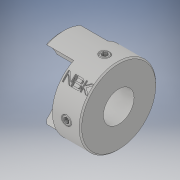
# Autodesk Inventor part: MJT-30-BL-8-12 Hub 2
Saved by Autodesk Inventor 2019 (Build 230136000, 136)
## iProperties
Created: 2023-09-29
Part Number: MJT-30-BL-8-12 Hub 2
Material: Generic
Catalog Web Link: www.cadenas.de
Description: MJT Hub 2-
Vendor: NBK
Document SubType Name: Modeling
Designer: psAdmin
Manufacturer: NBK
Mass: 7.813 g
Surface Area: 34.5036 cm^2
Volume: 7.813 cm^3
Density: 1 g/cm^3
Appearance: PSOLRGB-175-175-175
Category: PARTsolutions
Company: NBK
Title: MJT-30-BL-8-12 Hub 2
Author: Cadenas PARTsolutions
PSOL_IDENT_0: {$CADENAS_DATA/23d-libs/nbk/motion_control_parts/couplicon_mini/jaw_type/mjt/mjt_3.prj},187 {VTYP=3D
PSOL_IDENT_1: },{NB=MJT-30-BL-8-12 Hub 2},{LINA=MJT-30-BL-8-12 Hub 2},{NN=MJT Hub 2},{DATE=25.09.2023 00:41:45},{G
PSOL_IDENT_2: EOMDATE=30.03.2016 02:13:54},{VERSION=},{LINEID=30},{WBVAR=D1D2},{WBNUMERIC=}  {NB=MJT-30-BL-8-12 Hu
PSOL_IDENT_3: b 2},{LINA=MJT-30-BL-8-12 Hub 2},{KT=DUMMY},{CN=MJT-30-BL},{D1D2=8-12},{D1D2X1='6-6','6-6.35','6-7','
PSOL_IDENT_4: 6-8','6-9.525','6-10','6-11','6-12','6-14','6-15','6-16','6.35-6.35','6.35-7','6.35-8','6.35-9.525','
PSOL_IDENT_5: 6.35-10','6.35-11','6.35-12','6.35-14','6.35-15','6.35-16','7-7','7-8','7-9.525','7-10','7-11','7-12'
PSOL_IDENT_6: ,'7-14','7-15','7-16','8-8','8-9.525','8-10','8-11','8-12','8-14','8-15','8-16','9.525-9.525','9.525
PSOL_IDENT_7: -10','9.525-11','9.525-12','9.525-14','9.525-15','9.525-16','10-10','10-11','10-12','10-14','10-15','
PSOL_IDENT_8: 10-16','11-11','11-12','11-14','11-15','11-16','12-12','12-14','12-15','12-16','14-14','14-15','14-1
PSOL_IDENT_9: 6','15-15','15-16','16-16'},{VERS=1},{YV=0.5},{YU=1.0},{A=30},{L=11},{W=35},{B=10},{C=1.5},{F=5.5},{
PSOL_IDENT_10: M=M4},{KDMM=3.242},{NDM=4.00},{KDMV=3.141},{DV=7.00},{D1=8},{D2=12},{DP=13.22},{DP1=0.00},{RV=1.500}
PSOL_IDENT_11: ,{S=2.0}
NB: MJT-30-BL-8-12 Hub 2
NN: MJT Hub 2
NBSYN: $CN.-$D1D2. Hub 2
LINA: MJT-30-BL-8-12 Hub 2
CATALOG: NBK (Nabeya Bi-tech Kaisha
CN: MJT-30-BL
D1D2: 8-12
D1D2X1: '6-6','6-6.35','6-7','6-8','6-9.525','6-10','6-11','6-12','6-14','6-15','6-16','6.35-6.35','6.35-7','6.35-8','6.35-9.525','6.35-10','6.35-11','6.35-12','6.35-14','6.35-15','6.35-16','7-7','7-8','7-9.525','7-10','7-11','7-12','7-14','7-15','7-16','8-8','8-9.525','8-10','8-11','8-12','8-14','8-15','8-16','9.525-9.525','9.525-10','9.525-11','9.525-12','9.525-14','9.525-15','9.525-16','10-10','10-11','10-12','10-14','10-15','10-16','11-11','11-12','11-14','11-15','11-16','12-12','12-14','12-15','12-16','14-14','14-15','14-16','15-15','15-16','16-16'
VERS: 1
YV: 0.5
YU: 1
A: 30
L: 11
W: 35
B: 10
C: 1.5
F: 5.5
M: M4
KDMM: 3.242
NDM: 4
KDMV: 3.141
DV: 7
DP: 13.22
DP1: 0
RV: 1.5
S: 2
SUPPLIER: NBK
ARTICLENO: MJT-30-BL-8-12 Hub 2
BOMINFO: MJT-30-BL-8-12 Hub 2
CREATOR: CADENAS GmbH
Autodesk Inventor part; units mm, degrees
sketch "Sketch_1" plane through (0, 0, 0) normal (0, 1, 0) x (-1, 0, 0)
  line L0 (22.5, 0) -> (0, 0)
  line L1 (22.5, 14) -> (21.5, 15)
  line L2 (21.5, 15) -> (0.5, 15)
  line L3 (0.5, 15) -> (0, 14.5)
  line L4 (0, 14.5) -> (0, 6)
  line L5 (0, 6) -> (22.5, 6)
  line L6 (22.5, 6) -> (22.5, 14)
  constraints: 14 end point
revolve "Revolution1" add sketch "Sketch_1" angle 360 about axis through (-22.5, 0, 0) along (-1, 0, 0)
sketch "Sketch_2" plane through (-11, 0, 0) normal (1, 0, 0) x (0, 0, -1)
  arc A0 (-6.61, 13.4651) -> (-6.61, -13.4651) centre (0, 0) ccw
  arc A1 (-6.61, -13.4651) -> (-1.6525, -7.3157) centre (-17.0197, 0) ccw
  arc A2 (-1.6525, -7.3157) -> (1.6525, -7.3157) centre (0, 0) ccw
  arc A3 (1.6525, -7.3157) -> (6.61, -13.4651) centre (17.0197, 0) ccw
  arc A4 (6.61, -13.4651) -> (6.61, 13.4651) centre (0, 0) ccw
  arc A5 (6.61, 13.4651) -> (1.6525, 7.3157) centre (17.0197, 0) ccw
  arc A6 (1.6525, 7.3157) -> (-1.6525, 7.3157) centre (0, 0) ccw
  arc A7 (-1.6525, 7.3157) -> (-6.61, 13.4651) centre (-17.0197, 0) ccw
  constraints: 16 point on circle, 8 centre point
extrude "Extrusion1" cut sketch "Sketch_2" against normal blind 11.5
sketch "Sketch_7" plane through (0, 0, 0) normal (0, 1, 0) x (-1, 0, 0)
  line L0 (5.5, 0) -> (5.5, 15)
  line L1 (5.5, 15) -> (7.5, 15)
  line L2 (7.5, 15) -> (7.121, 14.621)
  line L3 (7.121, 14.621) -> (7.121, 0.379)
  line L4 (7.121, 0.379) -> (7.5, 0)
  line L5 (7.5, 0) -> (5.5, 0)
  line L6 (5.5, 0) -> (5.5, 15)
  constraints: 14 end point
revolve "Revolution2" cut sketch "Sketch_7" angle 360 about axis through (-5.5, 0, 0) along (0, 0, -1)
sketch "Sketch_8" plane through (0, 0, 0) normal (0, 0, 1) x (1, 0, 0)
  line L0 (-5.5, 15) -> (-5.5, 0)
  line L1 (-5.5, 0) -> (-7.5, 0)
  line L2 (-7.5, 0) -> (-7.121, 0.379)
  line L3 (-7.121, 0.379) -> (-7.121, 14.621)
  line L4 (-7.121, 14.621) -> (-7.5, 15)
  line L5 (-7.5, 15) -> (-5.5, 15)
  line L6 (-5.5, 15) -> (-5.5, 0)
  constraints: 14 end point
revolve "Revolution3" cut sketch "Sketch_8" angle 360 about axis through (-5.5, 15, 0) along (0, 1, 0)
sketch "Sketch_12" plane through (0, 0, 0) normal (0, 1, 0) x (-1, 0, 0)
  line L0 (5.5, 8) -> (5.5, 15)
  line L1 (5.5, 15) -> (7.0705, 15)
  line L2 (7.0705, 15) -> (7.5, 14.5705)
  line L3 (7.5, 14.5705) -> (7.5, 8.4295)
  line L4 (7.5, 8.4295) -> (7.0705, 8)
  line L5 (7.0705, 8) -> (5.5, 8)
  line L6 (5.5, 8) -> (5.5, 15)
  constraints: 14 end point
revolve "Revolution4" add sketch "Sketch_12" angle 360 about axis through (-5.5, 0, 8) along (0, 0, -1)
sketch "Sketch_13" plane through (0, 0, 0) normal (0, 0, 1) x (1, 0, 0)
  line L0 (-5.5, 15) -> (-5.5, 8)
  line L1 (-5.5, 8) -> (-7.0705, 8)
  line L2 (-7.0705, 8) -> (-7.5, 8.4295)
  line L3 (-7.5, 8.4295) -> (-7.5, 14.5705)
  line L4 (-7.5, 14.5705) -> (-7.0705, 15)
  line L5 (-7.0705, 15) -> (-5.5, 15)
  line L6 (-5.5, 15) -> (-5.5, 8)
  constraints: 14 end point
revolve "Revolution5" add sketch "Sketch_13" angle 360 about axis through (-5.5, 15, 0) along (0, 1, 0)
sketch "Sketch_14" plane through (0, 0, 13.5) normal (0, 0, 1) x (1, 0, 0)
  line L0 (-6.5, -0.5774) -> (-5.5, -1.1547)
  line L1 (-5.5, -1.1547) -> (-4.5, -0.5774)
  line L2 (-4.5, -0.5774) -> (-4.5, 0.5774)
  line L3 (-4.5, 0.5774) -> (-5.5, 1.1547)
  line L4 (-5.5, 1.1547) -> (-6.5, 0.5774)
  line L5 (-6.5, 0.5774) -> (-6.5, -0.5774)
  constraints: 12 end point
extrude "Extrusion2" cut sketch "Sketch_14" along normal blind 1.5
sketch "Sketch_15" plane through (0, 13.5, 0) normal (0, 1, 0) x (1, 0, 0)
  line L0 (-6.5, -0.5774) -> (-5.5, -1.1547)
  line L1 (-5.5, -1.1547) -> (-4.5, -0.5774)
  line L2 (-4.5, -0.5774) -> (-4.5, 0.5774)
  line L3 (-4.5, 0.5774) -> (-5.5, 1.1547)
  line L4 (-5.5, 1.1547) -> (-6.5, 0.5774)
  line L5 (-6.5, 0.5774) -> (-6.5, -0.5774)
  constraints: 12 end point
extrude "Extrusion3" cut sketch "Sketch_15" along normal blind 1.5
sketch "Sketch_19" plane through (0, 10.6066, 10.6066) normal (0, 0.7071, 0.7071) x (1, 0, 0)
  line L0 (-10.34, -1.815) -> (-9.79, -1.815)
  line L1 (-9.79, -1.815) -> (-9.79, 0.715)
  line L2 (-9.79, 0.715) -> (-7.7764, -1.6399)
  arc A0 (-7.7764, -1.6399) -> (-7.3963, -1.815) centre (-7.3963, -1.315) ccw
  line L3 (-7.3963, -1.815) -> (-7.0767, -1.815)
  line L4 (-7.0767, -1.815) -> (-7.0767, 1.815)
  line L5 (-7.0767, 1.815) -> (-7.6267, 1.815)
  line L6 (-7.6267, 1.815) -> (-7.6267, -0.715)
  line L7 (-7.6267, -0.715) -> (-9.6403, 1.6399)
  arc A1 (-9.6403, 1.6399) -> (-10.0203, 1.815) centre (-10.0203, 1.315) ccw
  line L8 (-10.0203, 1.815) -> (-10.34, 1.815)
  line L9 (-10.34, 1.815) -> (-10.34, -1.815)
  constraints: 20 end point, 4 point on circle, 2 centre point
sketch "Sketch_20" plane through (0, 10.6066, 10.6066) normal (0, 0.7071, 0.7071) x (1, 0, 0)
  line L0 (-6.8567, -1.815) -> (-4.5833, -1.815)
  arc A0 (-4.5833, -1.815) -> (-4.0386, 0.1218) centre (-4.5833, -0.77) ccw
  arc A1 (-4.0386, 0.1218) -> (-4.8583, 1.815) centre (-4.8583, 0.77) ccw
  line L1 (-4.8583, 1.815) -> (-6.8567, 1.815)
  line L2 (-6.8567, 1.815) -> (-6.8567, -1.815)
  line L3 (-6.3067, 0.275) -> (-4.8583, 0.275)
  arc A2 (-4.8583, 0.275) -> (-4.8583, 1.265) centre (-4.8583, 0.77) ccw
  line L4 (-4.8583, 1.265) -> (-6.3067, 1.265)
  line L5 (-6.3067, 1.265) -> (-6.3067, 0.275)
  line L6 (-6.3067, -1.265) -> (-4.5833, -1.265)
  arc A3 (-4.5833, -1.265) -> (-4.5833, -0.275) centre (-4.5833, -0.77) ccw
  line L7 (-4.5833, -0.275) -> (-6.3067, -0.275)
  line L8 (-6.3067, -0.275) -> (-6.3067, -1.265)
  constraints: 18 end point, 8 point on circle, 4 centre point
extrude "Extrusion4" cut sketch "Sketch_19" against normal blind 0.55
extrude "Extrusion5" cut sketch "Sketch_20" against normal blind 0.55
sketch "Sketch_21" plane through (0, 10.6066, 10.6066) normal (0, 0.7071, 0.7071) x (1, 0, 0)
  line L0 (-3.3733, -1.815) -> (-2.8233, -1.815)
  line L1 (-2.8233, -1.815) -> (-2.8233, -0.4614)
  line L2 (-2.8233, -0.4614) -> (-1.3633, -1.6863)
  arc A0 (-1.3633, -1.6863) -> (-1.0098, -1.815) centre (-1.0098, -1.265) ccw
  line L3 (-1.0098, -1.815) -> (-0.66, -1.815)
  line L4 (-0.66, -1.815) -> (-0.66, -1.265)
  line L5 (-0.66, -1.265) -> (-2.1678, 0)
  line L6 (-2.1678, 0) -> (-0.66, 1.265)
  line L7 (-0.66, 1.265) -> (-0.66, 1.815)
  line L8 (-0.66, 1.815) -> (-1.0098, 1.815)
  arc A1 (-1.0098, 1.815) -> (-1.3633, 1.6863) centre (-1.0098, 1.265) ccw
  line L9 (-1.3633, 1.6863) -> (-2.8233, 0.4614)
  line L10 (-2.8233, 0.4614) -> (-2.8233, 1.815)
  line L11 (-2.8233, 1.815) -> (-3.3733, 1.815)
  line L12 (-3.3733, 1.815) -> (-3.3733, -1.815)
  constraints: 26 end point, 4 point on circle, 2 centre point
extrude "Extrusion6" cut sketch "Sketch_21" against normal blind 0.55
ref_plane "part3_XY" through (-12.5, 0, 0) normal (1, 0, 0) x (0, 0, -1)
ref_plane "part3_YZ" through (-12.5, 0, 0) normal (0, 0, -1) x (0, 1, 0)
ref_plane "part3_ZX" through (-12.5, 0, 0) normal (0, 1, 0) x (1, 0, 0)
body "Solid1"
